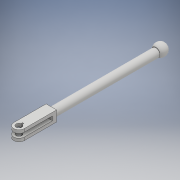
# Autodesk Inventor part: EndJoint
Saved by Autodesk Inventor 2018 (Build 220112000, 112)
## iProperties
Created: 2017-06-01
Part Number: EndJoint
Material: Generic
Document SubType Name: Modeling
Designer: Damian
Density: 1 g/cm^3
Appearance: Default
Author: Damian
Autodesk Inventor part; units mm, degrees
ref_plane "YZ Plane" through (0, 0, 0) normal (1, 0, 0) x (0, 1, 0)
ref_plane "XZ Plane" through (0, 0, 0) normal (0, 1, 0) x (-1, 0, 0)
ref_plane "XY Plane" through (0, 0, 0) normal (0, 0, 1) x (1, 0, 0)
sketch "Sketch1" plane through (0, 0, 0) normal (1, 0, 0) x (0, 1, 0)
  line L0 (0, 4.5) -> (36, 4.5)
  line L1 (36, 4.5) -> (36, -5.5)
  line L2 (36, -5.5) -> (0, -5.5)
  line L3 (0, -5.5) -> (0, -2.5)
  line L4 (0, -2.5) -> (32, -2.5)
  line L5 (32, -2.5) -> (32, 1.5)
  line L6 (32, 1.5) -> (0, 1.5)
  line L7 (0, 1.5) -> (0, 4.5)
  point P0 (0, 0)
  dimension "d0" = 3
  dimension "d1" = 32
  dimension "d2" = 4
  dimension "d3" = 4
  dimension "d11" = 2.5
  dimension "d12" = 0
  constraints: 16 end point, 7 perpendicular, 1 collinear, 1 horizontal, 1 point on line
  measures "d0" distance of L2.end L3.end
  measures "d1" distance of L3.end L4.end
  measures "d2" horizontal distance of L4.end L1.end
  measures "d3" distance of L4.end L5.end
  measures "d11" distance of L3.end point (0, 0)
  measures "d12" horizontal distance of point (0, 0) L3.end
extrude "Extrusion1" add sketch "Sketch1" along normal blind 10
sketch "Sketch2" plane through (0, 36, 4.5) normal (0, 1, 0) x (1, 0, 0)
  circle A0 centre (5, 5) radius 4
  line L0 (0, 0) -> (0, 10) projected
  line L1 (0, 10) -> (10, 10) projected
  point P0 (0, 4.5)
  dimension "d6" = 8
  dimension "d7" = 5
  dimension "d8" = 5
  constraints: 1 centre point
  measures "d6" diameter of A0
  measures "d7" distance from line of L0 A0.centre
  measures "d8" distance from line of L1 A0.centre
extrude "Extrusion2" add sketch "Sketch2" along normal blind 100
sketch "Sketch3" plane through (0, 0, 0) normal (0, 0, 1) x (1, 0, 0)
  line L0 (9, 136) -> (1, 136) projected
  line L1 (1, 136) -> (5, 136)
  line L2 (5, 136) -> (5, 146)
  arc A0 (5, 146) -> (1, 136) centre (5, 140.2) ccw
  point P0 (0, 0)
  dimension "d13" = 10
  constraints: 4 end point, 2 point on circle, 1 centre point, 1 midpoint, 1 perpendicular, 1 point on line
  measures "d13" distance of L1.end L2.end
revolve "Revolution1" add sketch "Sketch3" angle 360 about axis through (5, 136, 0) along (0, 1, 0)
fillet "Fillet1" radius 5 4 edges at (0, 0, -4) (10, 0, -4) (10, 0, 3) (0, 0, 3)
hole "Hole1" at (5, 5, -5.5) direction (0, 0, 1) diameter 5.5 end through all
sketch "Sketch4" plane through (10, 36, -5.5) normal (0, 0, -1) x (-1, 0, 0)
  circle A0 centre (5, -31) radius 2.75 projected
  line L0 (4.325, -28.3341) -> (4.325, -26.9841)
  line L1 (4.325, -26.9841) -> (5.675, -26.9841)
  line L2 (5.675, -26.9841) -> (5.675, -28.3341)
  line L3 (4.325, -28.3341) -> (5.675, -28.3341)
  point P0 (10, -36)
  dimension "d25" = 1.35
  dimension "d26" = 0.675
  dimension "d27" = 1.35
  constraints: 8 end point, 3 point on circle, 2 perpendicular, 1 horizontal, 1 vertical
  measures "d25" distance of L0.end L1.end
  measures "d26" horizontal distance of L0.start A0.centre
  measures "d27" distance of L1.end L2.end
extrude "Extrusion3" cut sketch "Sketch4" against normal through all contours A0 L0 L1 L2
body "Solid1"
